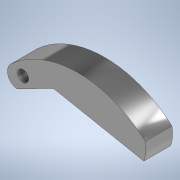
# Autodesk Inventor part: Peça 12
Saved by Autodesk Inventor 2021 (Build 250183000, 183)
## iProperties
Created: 2020-11-14
Part Number: Peça 12
Material: Liga de Nickel-Copper 400
Document SubType Name: Modeling
Designer: Bruno
Density: 8.83 g/cm^3
Appearance: Cromado - Preto polido
Author: Bruno
Autodesk Inventor part; units mm, degrees
ref_plane "YZ Plane" through (0, 0, 0) normal (1, 0, 0) x (0, 1, 0)
ref_plane "XZ Plane" through (0, 0, 0) normal (0, 1, 0) x (-1, 0, 0)
ref_plane "XY Plane" through (0, 0, 0) normal (0, 0, 1) x (1, 0, 0)
sketch "Esboço2" plane through (0, 0, 0) normal (0, 0, 1) x (1, 0, 0)
  arc A0 (3.02, 3.3361) -> (-3.02, 3.3361) centre (0, 0) ccw
  line L0 (-3.02, 3.3361) -> (3.02, 3.3361)
  line L1 (-1.1113, 3.3361) -> (2.9551, 2.5361)
  arc A1 (2.9551, 2.5361) -> (3.02, 3.3361) centre (1.6299, 3.0462) ccw
  line L2 (-1.1113, 3.3361) -> (-2.7507, 2.4931)
  arc A2 (-3.02, 3.3361) -> (-2.7507, 2.4931) centre (-2.6938, 2.9758) ccw
  dimension "d8" = 9
  dimension "d9" = 6.04
  dimension "d10" = 0.8
  dimension "d11" = 0.843
  constraints: 6 end point, 6 point on circle, 3 centre point, 1 coincident, 1 horizontal, 1 point on line, 1 tangent
  measures "d8" diameter of A0
  measures "d9" distance of L0.start L0.end
  measures "d10" vertical distance of L1.end L0.end
  measures "d11" vertical distance of L2.end L0.start
extrude "Extrusão1" add sketch "Esboço2" against normal blind 1.2
sketch "Esboço3" plane through (0, 0, 0) normal (0, 0, 1) x (1, 0, 0)
  circle A0 centre (-2.473, 3.141) radius 0.25
  line L0 (0, 5.4) -> (0, -0.9) projected
  line L1 (-4.4258, 0) -> (4.2958, 0) projected
  point P0 (0, 0)
  dimension "d14" = 0.5
  dimension "d16" = 2.473
  dimension "d17" = 3.141
  constraints: 1 centre point
  measures "d14" diameter of A0
  measures "d16" distance from line of L0 A0.centre
  measures "d17" distance from line of L1 A0.centre
extrude "Extrusão2" cut sketch "Esboço3" against normal through all
